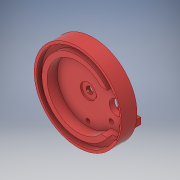
# Autodesk Inventor part: joint2_rotate_mec
Saved by Autodesk Inventor 2019 (Build 230136000, 136)
## iProperties
Created: 2019-12-26
Part Number: joint2_rotate_mec
Material: Пластик АБС
Document SubType Name: Modeling
Designer: Петров Иван
Density: 1.06 g/cm^3
Appearance: Гладкий — красный
Author: Петров Иван
Autodesk Inventor part; units mm, degrees
ref_plane "YZ Plane" through (0, 0, 0) normal (1, 0, 0) x (0, 1, 0)
ref_plane "XZ Plane" through (0, 0, 0) normal (0, 1, 0) x (-1, 0, 0)
ref_plane "XY Plane" through (0, 0, 0) normal (0, 0, 1) x (1, 0, 0)
sketch "Эскиз2" plane through (0, 0, 0) normal (0, 0, 1) x (1, 0, 0)
  circle A0 centre (0, 0) radius 42.5
  dimension "d0" = 85
  constraints: 1 centre point, 1 coincident
  measures "d0" diameter of A0
extrude "Выдавливание1" add sketch "Эскиз2" along normal blind 5
sketch "Эскиз3" plane through (0, 0, 5) normal (0, 0, 1) x (1, 0, 0)
  circle A0 centre (27.5, 0) radius 7
  arc A1 (22.4345, 19.9171) -> (22.4345, -19.9171) centre (0, 0) ccw
  line L0 (32.5655, -19.9171) -> (22.4345, -19.9171)
  arc A2 (32.5655, -19.9171) -> (38.9118, -17.0915) centre (27.5, 0) ccw
  arc A3 (38.9118, -17.0915) -> (37.5441, 19.9171) centre (0, 0) ccw
  line L1 (22.4345, 19.9171) -> (37.5441, 19.9171)
  circle A4 centre (32.45, -14.15) radius 2.15
  circle A5 centre (0, 0) radius 8
  circle A6 centre (22.55, -14.15) radius 2.15
  arc A7 (32.5655, -19.9171) -> (38.9118, -17.0915) centre (27.5, 0) ccw
  line L2 (32.5655, -19.9171) -> (22.4345, -19.9171)
  arc A8 (22.4345, 19.9171) -> (22.4345, -19.9171) centre (0, 0) ccw
  line L3 (22.4345, 19.9171) -> (37.5441, 19.9171)
  arc A9 (37.5441, 19.9171) -> (38.9118, -17.0915) centre (0, 0) ccw
  point P0 (0, -36.1)
  constraints: 12 point on circle, 10 centre point, 8 end point
extrude "Выдавливание2" add sketch "Эскиз3" along normal blind 10 contours A1 L0 A2 A9 L1
sketch "Эскиз4" plane through (0, 0, 5) normal (0, 0, 1) x (1, 0, 0)
  circle A0 centre (27.5, 0) radius 7
  arc A1 (22.4345, 19.9171) -> (22.4345, -19.9171) centre (0, 0) ccw
  line L0 (32.5655, -19.9171) -> (22.4345, -19.9171)
  arc A2 (32.5655, -19.9171) -> (38.9118, -17.0915) centre (27.5, 0) ccw
  arc A3 (38.9118, -17.0915) -> (37.5441, 19.9171) centre (0, 0) ccw
  line L1 (22.4345, 19.9171) -> (37.5441, 19.9171)
  circle A4 centre (32.45, -14.15) radius 2.15
  circle A5 centre (0, 0) radius 8
  circle A6 centre (22.55, -14.15) radius 2.15
  arc A7 (32.5655, -19.9171) -> (38.9118, -17.0915) centre (27.5, 0) ccw
  line L2 (32.5655, -19.9171) -> (22.4345, -19.9171)
  arc A8 (22.4345, 19.9171) -> (22.4345, -19.9171) centre (0, 0) ccw
  line L3 (22.4345, 19.9171) -> (37.5441, 19.9171)
  arc A9 (37.5441, 19.9171) -> (38.9118, -17.0915) centre (0, 0) ccw
  point P0 (0, -36.1)
  constraints: 12 point on circle, 10 centre point, 8 end point
extrude "Выдавливание3" cut sketch "Эскиз4" against normal blind 10 contours A0 | A4 | A5 | A6
sketch "Эскиз5" plane through (-19.7699, -0.8287, 0) normal (0, 0, -1) x (-1, 0, 0)
  line L0 (-37.2699, -9.1713) -> (-57.2699, -9.1713)
  line L1 (-57.2699, -9.1713) -> (-57.2699, -15.1713)
  arc A0 (-57.2699, -15.1713) -> (-56.2699, -16.1713) centre (-56.2699, -15.1713) ccw
  line L2 (-56.2699, -16.1713) -> (-53.4199, -16.1713)
  arc A1 (-51.0199, -15.1052) -> (-53.4199, -15.1052) centre (-52.2199, -13.3213) ccw
  line L3 (-51.0199, -16.1713) -> (-43.5199, -16.1713)
  arc A2 (-41.1199, -15.1052) -> (-43.5199, -15.1052) centre (-42.3199, -13.3213) ccw
  line L4 (-41.1199, -16.1713) -> (-38.2699, -16.1713)
  arc A3 (-38.2699, -16.1713) -> (-37.2699, -15.1713) centre (-38.2699, -15.1713) ccw
  line L5 (-37.2699, -15.1713) -> (-37.2699, -9.1713)
  line L6 (-43.5199, 38.5287) -> (-43.5199, 37.4627)
  line L7 (-51.0199, 38.5287) -> (-43.5199, 38.5287)
  line L8 (-51.0199, 37.4627) -> (-51.0199, 38.5287)
  arc A4 (-53.4199, 37.4627) -> (-51.0199, 37.4627) centre (-52.2199, 35.6787) ccw
  line L9 (-53.4199, 38.5287) -> (-53.4199, 37.4627)
  line L10 (-56.2699, 38.5287) -> (-53.4199, 38.5287)
  arc A5 (-56.2699, 38.5287) -> (-57.2699, 37.5287) centre (-56.2699, 37.5287) ccw
  line L11 (-57.2699, 31.5287) -> (-57.2699, 37.5287)
  line L12 (-37.2699, 31.5287) -> (-57.2699, 31.5287)
  line L13 (-37.2699, 37.5287) -> (-37.2699, 31.5287)
  arc A6 (-37.2699, 37.5287) -> (-38.2699, 38.5287) centre (-38.2699, 37.5287) ccw
  line L14 (-41.1199, 38.5287) -> (-38.2699, 38.5287)
  line L15 (-41.1199, 37.4627) -> (-41.1199, 38.5287)
  arc A7 (-43.5199, 37.4627) -> (-41.1199, 37.4627) centre (-42.3199, 35.6787) ccw
  line L16 (-57.2699, -9.1713) -> (-57.2699, 31.5287)
  line L17 (-37.2699, 31.5287) -> (-37.2699, -9.1713)
  line L18 (-37.2699, -9.1713) -> (-57.2699, -9.1713)
  circle A8 centre (-47.2699, 0.8287) radius 1.25
  circle A9 centre (-47.2699, 0.8287) radius 3.4957
  circle A10 centre (-47.2699, 0.8287) radius 2.6787
  circle A11 centre (-47.2699, 0.8287) radius 5.4
  line L19 (-37.2699, -14.1713) -> (-37.2699, 15.8287)
  line L20 (-37.2699, 0.8287) -> (-47.2699, 0.8287)
  circle A12 centre (-52.2199, -13.3213) radius 2.15
  circle A13 centre (-42.3199, -13.3213) radius 2.15
  line L21 (-53.4199, -16.1713) -> (-51.0199, -16.1713)
  line L22 (-43.5199, -16.1713) -> (-40.9117, -16.1713)
  circle A14 centre (-52.2199, -13.3213) radius 2.15 projected
  point P0 (0, -36.1)
  point P1 (0, -36.1)
  point P2 (-37.2699, 11.1787)
  dimension "d7" = 10
  constraints: 46 end point, 16 point on circle, 14 centre point, 2 coincident, 2 concentric, 2 horizontal, 1 midpoint, 1 point on line
  measures "d7" distance of L20.start L20.end
extrude "Выдавливание4" add sketch "Эскиз5" along normal blind 8.6 contours L5 A3 L4 L22 L3 L21 L2 A0 L1 L0
sketch "Эскиз6" plane through (0, 0, 5) normal (0, 0, 1) x (1, 0, 0)
  circle A0 centre (0, 25) radius 1.9
  circle A1 centre (0, -25) radius 1.9
  circle A2 centre (0, 0) radius 8
  line L0 (-17.5, -36.1) -> (17.5, -36.1)
  line L1 (17.5, -36.1) -> (17.5, 36.1)
  line L2 (17.5, 36.1) -> (-17.5, 36.1)
  line L3 (-17.5, 36.1) -> (-17.5, -36.1)
  point P0 (0, -36.1)
  constraints: 8 end point, 3 centre point
extrude "Выдавливание5" cut sketch "Эскиз6" against normal blind 10 contours A0 | A1
sketch "Эскиз7" plane through (0, 0, 5) normal (0, 0, 1) x (1, 0, 0)
  point P0 (0, 0)
sketch "Эскиз8" plane through (0, 0, 5) normal (0, 0, 1) x (1, 0, 0)
  circle A0 centre (0, 0) radius 8
  circle A1 centre (0, 0) radius 5.375
  circle A2 centre (0, 0) radius 3.375
  line L0 (-6.9327, -1) -> (-6.9327, 1)
  line L1 (-8.2327, 1.5) -> (-6.9327, 1.5)
  line L2 (-6.9327, -1.5) -> (-6.9327, -1)
  line L3 (-6.9327, -1.5) -> (-8.2327, -1.5)
  spline S0 degree 3 poles (-8.2327, -1.5) (-8.2334, -1.4968) (-8.234, -1.4935) (-8.2347, -1.4903) (-8.2347, -1.4901) (-8.2347, -1.49) (-8.2361, -1.4829) (-8.2382, -1.4724) (-8.2457, -1.4333) (-8.2525, -1.3974) (-8.2687, -1.3062) (-8.278, -1.2509) (-8.2965, -1.1299) (-8.3056, -1.0653) (-8.3138, -1) knots 0 0 0 0 0.066869 0.066869 0.066869 0.069411 0.069411 0.210348 0.210348 0.466356 0.466356 0.734146 0.734146 1 1 1 1
  ellipse E0 centre (-0.8138, 2.2378) end of major axis (-6.2384, -4.8493) minor radius 6.6293 (-8.308, 1) -> (-8.3138, -1) ccw
  spline S1 degree 3 poles (-8.308, 1) (-8.3, 1.0653) (-8.2914, 1.1299) (-8.274, 1.2508) (-8.2654, 1.3061) (-8.2506, 1.3973) (-8.2444, 1.4332) (-8.2376, 1.4723) (-8.2358, 1.4829) (-8.2345, 1.49) (-8.2345, 1.4901) (-8.2345, 1.4902) (-8.2339, 1.4935) (-8.2333, 1.4967) (-8.2327, 1.5) knots 0 0 0 0 0.265855 0.265855 0.533308 0.533308 0.789424 0.789424 0.930547 0.930547 0.932946 0.932946 0.932946 1 1 1 1
  dimension "d18" = 6.75
  constraints: 8 end point, 3 centre point, 1 coincident, 8 other
  measures "d18" diameter of A2
extrude "Выдавливание6" add sketch "Эскиз8" against normal blind 5 contours A0 | A1
sketch "Эскиз9" plane through (0, 0, 0) normal (0, 0, -1) x (-1, 0, 0)
  circle A0 centre (0, 0) radius 8
  circle A1 centre (0, 0) radius 5.375
  circle A2 centre (0, 0) radius 3.375
  line L0 (-6.9327, -1) -> (-6.9327, 1)
  line L1 (-8.2327, 1.5) -> (-6.9327, 1.5)
  line L2 (-6.9327, -1.5) -> (-6.9327, -1)
  line L3 (-6.9327, -1.5) -> (-8.2327, -1.5)
  spline S0 degree 3 poles (-8.2327, -1.5) (-8.2334, -1.4968) (-8.234, -1.4935) (-8.2347, -1.4903) (-8.2347, -1.4901) (-8.2347, -1.49) (-8.2361, -1.4829) (-8.2382, -1.4724) (-8.2457, -1.4333) (-8.2525, -1.3974) (-8.2687, -1.3062) (-8.278, -1.2509) (-8.2965, -1.1299) (-8.3056, -1.0653) (-8.3138, -1) knots 0 0 0 0 0.066869 0.066869 0.066869 0.069411 0.069411 0.210348 0.210348 0.466356 0.466356 0.734146 0.734146 1 1 1 1
  ellipse E0 centre (-0.8138, 2.2378) end of major axis (-6.2384, -4.8493) minor radius 6.6293 (-8.308, 1) -> (-8.3138, -1) ccw
  spline S1 degree 3 poles (-8.308, 1) (-8.3, 1.0653) (-8.2914, 1.1299) (-8.274, 1.2508) (-8.2654, 1.3061) (-8.2506, 1.3973) (-8.2444, 1.4332) (-8.2376, 1.4723) (-8.2358, 1.4829) (-8.2345, 1.49) (-8.2345, 1.4901) (-8.2345, 1.4902) (-8.2339, 1.4935) (-8.2333, 1.4967) (-8.2327, 1.5) knots 0 0 0 0 0.265855 0.265855 0.533308 0.533308 0.789424 0.789424 0.930547 0.930547 0.932946 0.932946 0.932946 1 1 1 1
  line L4 (-6.9327, 1.5) -> (-8.5461, 1.5)
  line L5 (-8.5461, 1.5) -> (-8.5461, -1.5)
  line L6 (-8.5461, -1.5) -> (-6.9327, -1.5)
  line L7 (-6.9327, -1.5) -> (-6.9327, 1.5)
  dimension "d19" = 6.75
  constraints: 16 end point, 3 centre point, 2 parallel, 1 coincident, 1 horizontal, 1 perpendicular, 8 other
  measures "d19" diameter of A2
extrude "Выдавливание7" cut sketch "Эскиз9" against normal blind 5 contours L1 L7 L0 L2 L3 A0 | A0 L3 S0 E0 S1 L1 | S1 E0 S0 L6 L5 L4 picked at (-7.2832, -0.1675)
sketch "Эскиз10" plane through (0, 0, 5) normal (0, 0, 1) x (1, 0, 0)
  arc A0 (32.5655, -19.9171) -> (38.9118, -17.0915) centre (27.5, 0) ccw projected
  line L0 (37.5441, 19.9171) -> (22.4345, 19.9171) projected
  arc A1 (37.3765, -18.0051) -> (35.8053, 19.9171) centre (-0.4631, -0.5792) ccw
  arc A2 (37.3765, -18.0051) -> (38.9118, -17.0915) centre (30.7338, -5.0939) ccw
  line L1 (37.4224, 19.9171) -> (35.8053, 19.9171)
  arc A3 (38.9118, -17.0915) -> (37.5441, 19.9171) centre (0, 0) ccw projected
  arc A4 (38.9118, -17.0915) -> (37.5441, 19.9171) centre (0, 0) ccw
  line L2 (37.5441, 19.9171) -> (35.8053, 19.9171)
  constraints: 6 point on circle, 4 end point, 3 centre point, 2 point on line, 1 collinear, 1 horizontal
extrude "Выдавливание8" add sketch "Эскиз10" along normal up to surface (10 mm away)
sketch "Эскиз11" plane through (0, 0, 15) normal (0, 0, 1) x (1, 0, 0)
  circle A0 centre (0, 0) radius 3.375 projected
  circle A1 centre (0, 0) radius 40
  circle A2 centre (0, 0) radius 35
  dimension "d25" = 80
  dimension "d26" = 70
  constraints: 2 centre point, 2 coincident
  measures "d25" diameter of A1
  measures "d26" diameter of A2
extrude "Выдавливание9" cut sketch "Эскиз11" against normal blind 5 contours A1
sketch "Эскиз12" plane through (0, 0, 5) normal (0, 0, 1) x (1, 0, 0)
  circle A0 centre (0, 0) radius 7.5
  dimension "d29" = 15
  constraints: 1 centre point, 1 coincident
  measures "d29" diameter of A0
extrude "Выдавливание10" cut sketch "Эскиз12" against normal blind 1.5
sketch "Эскиз13" plane through (0, 0, 15) normal (0, 0, 1) x (1, 0, 0)
  circle A0 centre (0, 0) radius 3.375 projected
  circle A1 centre (0, 0) radius 44
  circle A2 centre (0.6251, 46.3721) radius 3.6178
  circle A3 centre (0.6251, 46.3721) radius 3.0311
  circle A4 centre (0.6251, 46.3721) radius 3.8133
  circle A5 centre (0.6251, 46.3721) radius 2.8356
  circle A6 centre (0.6251, 46.3721) radius 1.9556
  circle A7 centre (0, 0) radius 42.5
  dimension "d32" = 88
  constraints: 7 centre point, 2 coincident
  measures "d32" diameter of A1
extrude "Выдавливание11" [suppressed]
sketch "Эскиз14" plane through (0, 0, 0) normal (0, 0, -1) x (-1, 0, 0)
  circle A0 centre (0, 0) radius 44
  circle A1 centre (0, 0) radius 42.5
  dimension "d35" = 85
  constraints: 2 centre point, 2 coincident
  measures "d35" diameter of A1
extrude "Выдавливание12" [suppressed]
